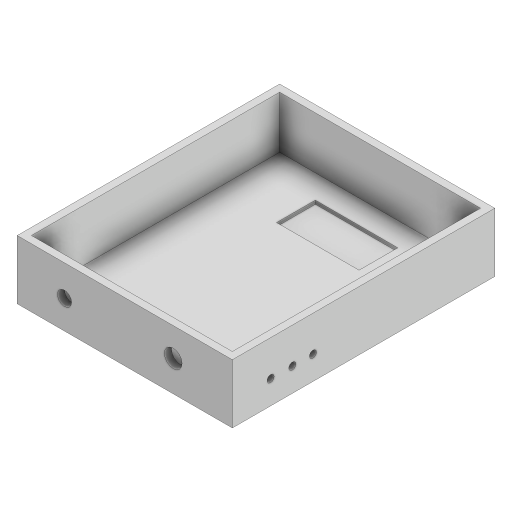
# Autodesk Inventor part: Caixa
Saved by Autodesk Inventor 2024.3 (Build 283343000, 343)
## iProperties
Created: 2023-08-31
Part Number: Caixa
Material: Genérico
Document SubType Name: Modeling
Designer: barof
Density: 1 g/cm^3
Appearance: Padrão
Author: barof
## iProperties of the stored document Caixa_3DPrint.ipt
Created: 2023-09-01
Part Number: Caixa_3DPrint
Material: Genérico
Document SubType Name: Modeling
Designer: barof
Density: 1 g/cm^3
Appearance: Padrão
Author: barof
Autodesk Inventor part; units mm, degrees
ref_plane "YZ Plane" through (0, 0, 0) normal (1, 0, 0) x (0, 1, 0)
ref_plane "XZ Plane" through (0, 0, 0) normal (0, 1, 0) x (-1, 0, 0)
ref_plane "XY Plane" through (0, 0, 0) normal (0, 0, 1) x (1, 0, 0)
sketch "Esboço1" plane through (0, 0, 0) normal (0, 1, 0) x (-1, 0, 0)
  line L0 (0, 0) -> (-91, 0)
  line L1 (-91, 0) -> (-91, -111)
  line L2 (-91, -111) -> (0, -111)
  line L3 (0, -111) -> (0, 0)
  line L4 (-3, -108) -> (-88, -108)
  line L5 (-88, -108) -> (-88, -3)
  line L6 (-88, -3) -> (-3, -3)
  line L7 (-3, -3) -> (-3, -108)
  dimension "d0" = 3
  dimension "d1" = 3
  dimension "d2" = 3
  dimension "d3" = 3
  dimension "d4" = 85
  dimension "d5" = 105
  constraints: 16 end point, 4 parallel, 2 horizontal, 2 perpendicular
  measures "d0" distance between parallel lines of L1 L5
  measures "d1" distance between parallel lines of L2 L4
  measures "d2" distance between parallel lines of L7 L3
  measures "d3" distance between parallel lines of L0 L6
  measures "d4" distance of L4.start L4.end
  measures "d5" distance of L4.end L5.end
extrude "Extrusão1" add sketch "Esboço1" along normal blind 3 contours L4 L5 L6 L7
extrude "Extrusão2" add sketch "Esboço1" along normal blind 25
sketch "Esboço2" plane through (0, 0, 0) normal (0, 0, 1) x (1, 0, 0)
  circle A0 centre (20, 12) radius 3
  circle A1 centre (66, 13) radius 3.75
  line L0 (0, 0) -> (0, 25) projected
  line L1 (91, 0) -> (91, 25) projected
  line L2 (0, 0) -> (91, 0) projected
  point P0 (0, 12.5)
  dimension "d10" = 6
  dimension "d11" = 7.5
  dimension "d25" = 20
  dimension "d26" = 25
  dimension "d30" = 13
  dimension "d31" = 12
  constraints: 2 centre point, 1 midpoint
  measures "d10" diameter of A0
  measures "d11" diameter of A1
  measures "d25" horizontal distance of point (0, 12.5) A0.centre
  measures "d26" distance from line of L1 A1.centre
  measures "d30" distance from line of A1.centre L2
  measures "d31" distance from line of A0.centre L2
extrude "Extrusão3" cut sketch "Esboço2" against normal blind 30
sketch "Esboço3" plane through (91, 0, 0) normal (1, 0, 0) x (0, 0, -1)
  circle A0 centre (16.1671, 10) radius 1.5
  circle A1 centre (34.0898, 10) radius 1.5
  circle A2 centre (25.3707, 10) radius 1.5
  line L0 (0, 0) -> (111, 0) projected
  dimension "d14" = 3
  dimension "d15" = 3
  dimension "d16" = 3
  dimension "d32" = 10
  dimension "d33" = 10
  dimension "d34" = 10
  constraints: 3 centre point
  measures "d14" diameter of A0
  measures "d15" diameter of A1
  measures "d16" diameter of A2
  measures "d32" distance from line of A0.centre L0
  measures "d33" distance from line of L0 A2.centre
  measures "d34" distance from line of L0 A1.centre
extrude "Extrusão4" cut sketch "Esboço3" against normal blind 10
sketch "Esboço4" plane through (0, 3, 0) normal (0, 1, 0) x (1, 0, 0)
  line L0 (28.1, 81.6) -> (63, 81.6)
  line L1 (63, 81.6) -> (63, 98)
  line L2 (63, 98) -> (28.1, 98)
  line L3 (28.1, 98) -> (28.1, 81.6)
  line L4 (88, 108) -> (88, 3) projected
  line L5 (3, 108) -> (88, 108) projected
  point P0 (0, 0)
  point P1 (63, 89.8)
  dimension "d19" = 34.9
  dimension "d20" = 16.4
  dimension "d23" = 25
  dimension "d24" = 10
  constraints: 8 end point, 2 parallel, 1 horizontal, 1 midpoint, 1 perpendicular
  measures "d19" distance of L2.end L1.end
  measures "d20" distance of L1.end L0.end
  measures "d23" distance from line of point (63, 89.8) L4
  measures "d24" distance between parallel lines of L5 L2
extrude "Extrusão5" cut sketch "Esboço4" against normal blind 1.5
